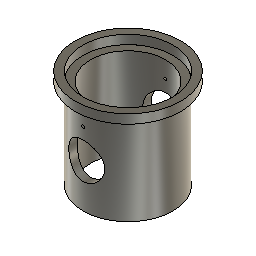
Injector assembly v3 (Autodesk Fusion 360 design; units mm, degrees)
Autodesk Fusion 360 part; units mm, degrees
sketch "Sketch1" plane through (0, 0, 0) normal (0, 0, 1) x (1, 0, 0)
  circle A0 centre (0, 0) radius 150.0959
  constraint coincident A0.centre origin
extrude "Extrude1" add sketch "Sketch1" along normal blind 300 makes body 1
hole "Hole1" at (0, 150.0959, 145.2237) direction (0, -1, 0) diameter 120 depth 340 tip angle 180 countersink diameter 132 countersink angle 90 bodies 1
hole "Hole2" at (0, 0, 300) direction (0, 0, -1) diameter 250 depth 300 tip angle 180 bodies 1
hole "Hole3" at (0, 150.0959, 244.2292) direction (0, -1, 0) diameter 10 depth 300 tip angle 180 bodies 1
sketch "Sketch2" plane through (0, 0, 300) normal (0, 0, 1) x (-1, 0, 0)
  circle A0 centre (0, 0) radius 125
  circle A1 centre (0, 0) radius 150.0959
  circle A2 centre (0, 0) radius 175.4784
  constraint coincident A0.centre A1.centre
extrude "Extrude2" add sketch "Sketch2" along normal blind 30 separate body contours A2 makes body 2
